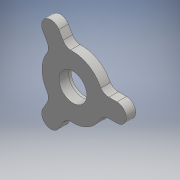
# Autodesk Inventor part: ET1
Saved by Autodesk Inventor 2016 (Build 200138000, 138)
## iProperties
Created: 2016-03-19
Part Number: ET1
Material: Genérico
Document SubType Name: Modeling
Designer: Usuario1
Density: 1 g/cm^3
Appearance: Valor por defecto
Author: Usuario1
Autodesk Inventor part; units mm, degrees
ref_plane "YZ Plane" through (0, 0, 0) normal (1, 0, 0) x (0, 1, 0)
ref_plane "XZ Plane" through (0, 0, 0) normal (0, 1, 0) x (-1, 0, 0)
ref_plane "XY Plane" through (0, 0, 0) normal (0, 0, 1) x (1, 0, 0)
sketch "Boceto1" plane through (0, 0, 0) normal (0, 1, 0) x (-1, 0, 0)
  arc A0 (-2.5488, 0.5326) -> (-2.5488, -0.5326) centre (-2.5488, 0) ccw
  circle A1 centre (-2.5488, 0) radius 0.2
  arc A2 (1.7357, 1.941) -> (0.8131, 2.4736) centre (1.2744, 2.2073) ccw
  circle A3 centre (1.2744, 2.2073) radius 0.2
  line L0 (-2.5488, 0.5326) -> (-2.2825, 0.5326)
  line L1 (-2.5488, -0.5326) -> (-2.2825, -0.5326)
  line L2 (0.8131, 2.4736) -> (0.6799, 2.243)
  line L3 (1.7357, 1.941) -> (1.6025, 1.7103)
  arc A4 (0.8131, -2.4736) -> (1.7357, -1.941) centre (1.2744, -2.2073) ccw
  circle A5 centre (1.2744, -2.2073) radius 0.2
  line L4 (1.7357, -1.941) -> (1.4977, -1.5289)
  arc A6 (1.4642, -1.0203) -> (1.4977, -1.5289) centre (1.9968, -1.2406) ccw
  circle A7 centre (0, 0) radius 0.8
  circle A8 centre (0, 0) radius 1.2
  arc A9 (0.5752, -2.0615) -> (0.1515, -1.7782) centre (0.076, -2.3496) ccw
  line L5 (0.5752, -2.0615) -> (0.8131, -2.4736)
  line L6 (-2.5488, -0.5326) -> (-2.0728, -0.5327)
  arc A10 (-1.6158, -0.7579) -> (-2.0728, -0.5327) centre (-2.0728, -1.109) ccw
  arc A11 (-2.0729, 0.5326) -> (-1.6158, 0.7579) centre (-2.0728, 1.109) ccw
  line L7 (-2.0729, 0.5326) -> (-2.5488, 0.5326)
  line L8 (0.8131, 2.4736) -> (0.5752, 2.0615)
  arc A12 (0.1515, 1.7782) -> (0.5752, 2.0615) centre (0.076, 2.3496) ccw
  arc A13 (1.4977, 1.5289) -> (1.4642, 1.0203) centre (1.9968, 1.2406) ccw
  line L9 (1.4977, 1.5289) -> (1.7357, 1.941)
  arc A14 (-1.6158, -0.7579) -> (0.1515, -1.7782) centre (0, 0) ccw
  arc A15 (0.1515, 1.7782) -> (-1.6158, 0.7579) centre (0, 0) ccw
  arc A16 (1.4642, -1.0203) -> (1.4642, 1.0203) centre (0, 0) ccw
  point P0 (0, 0)
  constraints: 24 point on circle, 20 end point, 17 centre point, 4 point on line
extrude "Extrusión1" add sketch "Boceto1" along normal blind 0.55 contours L0 L7 A11 A15 A12 L8 L2 A2 L3 L9 A13 A16 A6 L4 A4 L5 A9 A14 A10 L6 L1 A0 | A8
sketch "Boceto2" plane through (0, 0.55, 0) normal (0, 1, 0) x (1, 0, 0)
  arc A0 (2.5488, -0.5326) -> (2.5488, 0.5326) centre (2.5488, 0) ccw
  circle A1 centre (2.5488, 0) radius 0.2
  arc A2 (-1.7357, -1.941) -> (-0.8131, -2.4736) centre (-1.2744, -2.2073) ccw
  circle A3 centre (-1.2744, -2.2073) radius 0.2
  line L0 (2.5488, -0.5326) -> (2.2825, -0.5326)
  line L1 (2.5488, 0.5326) -> (2.2825, 0.5326)
  line L2 (-0.8131, -2.4736) -> (-0.6799, -2.243)
  line L3 (-1.7357, -1.941) -> (-1.6025, -1.7103)
  arc A4 (-0.8131, 2.4736) -> (-1.7357, 1.941) centre (-1.2744, 2.2073) ccw
  circle A5 centre (-1.2744, 2.2073) radius 0.2
  line L4 (-1.7357, 1.941) -> (-1.4977, 1.5289)
  arc A6 (-1.4642, 1.0203) -> (-1.4977, 1.5289) centre (-1.9968, 1.2406) ccw
  circle A7 centre (0, 0) radius 0.8
  circle A8 centre (0, 0) radius 1.2
  arc A9 (-0.5752, 2.0615) -> (-0.1515, 1.7782) centre (-0.076, 2.3496) ccw
  line L5 (-0.5752, 2.0615) -> (-0.8131, 2.4736)
  line L6 (2.5488, 0.5326) -> (2.0728, 0.5327)
  arc A10 (1.6158, 0.7579) -> (2.0728, 0.5327) centre (2.0728, 1.109) ccw
  arc A11 (2.0728, -0.5326) -> (1.6158, -0.7579) centre (2.0728, -1.109) ccw
  line L7 (2.0728, -0.5326) -> (2.5488, -0.5326)
  line L8 (-0.8131, -2.4736) -> (-0.5752, -2.0615)
  arc A12 (-0.1515, -1.7782) -> (-0.5752, -2.0615) centre (-0.076, -2.3496) ccw
  arc A13 (-1.4977, -1.5289) -> (-1.4642, -1.0203) centre (-1.9968, -1.2406) ccw
  line L9 (-1.4977, -1.5289) -> (-1.7357, -1.941)
  arc A14 (1.6158, 0.7579) -> (-0.1515, 1.7782) centre (0, 0) ccw
  arc A15 (-0.1515, -1.7782) -> (1.6158, -0.7579) centre (0, 0) ccw
  arc A16 (-1.4642, 1.0203) -> (-1.4642, -1.0203) centre (0, 0) ccw
  constraints: 24 point on circle, 20 end point, 17 centre point, 4 point on line
extrude "Extrusión2" add sketch "Boceto2" along normal blind 0.15 contours A8
sketch "Boceto3" plane through (0, 0, 0) normal (0, 1, 0) x (-1, 0, 0)
  arc A0 (-2.5488, 0.5326) -> (-2.5488, -0.5326) centre (-2.5488, 0) ccw
  circle A1 centre (-2.5488, 0) radius 0.2
  arc A2 (1.7357, 1.941) -> (0.8131, 2.4736) centre (1.2744, 2.2073) ccw
  circle A3 centre (1.2744, 2.2073) radius 0.2
  line L0 (-2.5488, 0.5326) -> (-2.2825, 0.5326)
  line L1 (-2.5488, -0.5326) -> (-2.2825, -0.5326)
  line L2 (0.8131, 2.4736) -> (0.6799, 2.243)
  line L3 (1.7357, 1.941) -> (1.6025, 1.7103)
  arc A4 (0.8131, -2.4736) -> (1.7357, -1.941) centre (1.2744, -2.2073) ccw
  circle A5 centre (1.2744, -2.2073) radius 0.2
  line L4 (1.7357, -1.941) -> (1.4977, -1.5289)
  arc A6 (1.4642, -1.0203) -> (1.4977, -1.5289) centre (1.9968, -1.2406) ccw
  circle A7 centre (0, 0) radius 0.8
  circle A8 centre (0, 0) radius 1.2
  arc A9 (0.5752, -2.0615) -> (0.1515, -1.7782) centre (0.076, -2.3496) ccw
  line L5 (0.5752, -2.0615) -> (0.8131, -2.4736)
  line L6 (-2.5488, -0.5326) -> (-2.0728, -0.5327)
  arc A10 (-1.6158, -0.7579) -> (-2.0728, -0.5327) centre (-2.0728, -1.109) ccw
  arc A11 (-2.0729, 0.5326) -> (-1.6158, 0.7579) centre (-2.0728, 1.109) ccw
  line L7 (-2.0729, 0.5326) -> (-2.5488, 0.5326)
  line L8 (0.8131, 2.4736) -> (0.5752, 2.0615)
  arc A12 (0.1515, 1.7782) -> (0.5752, 2.0615) centre (0.076, 2.3496) ccw
  arc A13 (1.4977, 1.5289) -> (1.4642, 1.0203) centre (1.9968, 1.2406) ccw
  line L9 (1.4977, 1.5289) -> (1.7357, 1.941)
  arc A14 (-1.6158, -0.7579) -> (0.1515, -1.7782) centre (0, 0) ccw
  arc A15 (0.1515, 1.7782) -> (-1.6158, 0.7579) centre (0, 0) ccw
  arc A16 (1.4642, -1.0203) -> (1.4642, 1.0203) centre (0, 0) ccw
  point P0 (0, 0)
  constraints: 24 point on circle, 20 end point, 17 centre point, 4 point on line
extrude "Extrusión3" add sketch "Boceto3" along normal blind 0.2 contours A1 | A3 | A5
